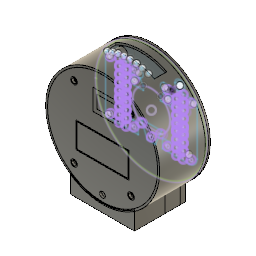
Whatscup design v30 (Autodesk Fusion 360 design; units mm, degrees)
Autodesk Fusion 360 part; units mm, degrees
note: some values were not read from the file. Chosen so that the rebuilt part matches the saved one: which face or edge a step refers to; which pieces of a blend or face edit are solid. Set by a fixed rule: which sketch regions a step uses.
(part 1 of 3)
sketch "Blueprint" plane through (0, 0, 0) normal (0, 1, 0) x (1, 0, 0)
  circle A0 centre (0, 0) radius 17.9
  line L0 (-5.49936, -34.775052) -> (17.60064, -34.775052)
  line L1 (17.60064, -34.775052) -> (17.60064, -22.275052)
  line L2 (17.60064, -22.275052) -> (-5.49936, -22.275052)
  line L3 (-5.49936, -22.275052) -> (-5.49936, -34.775052)
  line L4 (-5.49936, -34.775052) -> (0.00064, -34.775052)
  line L5 (0.00064, -34.775052) -> (0.00064, -22.275052)
  line L6 (0.00064, -22.275052) -> (-5.49936, -22.275052)
  line L7 (-5.49936, -22.275052) -> (-5.49936, -34.775052)
  line L8 (-31.404883, 42.880454) -> (31.412157, 42.880454)
  line L9 (31.412157, 42.880454) -> (31.412157, 63.421004)
  line L10 (31.412157, 63.421004) -> (-31.404883, 63.421004)
  line L11 (-31.404883, 63.421004) -> (-31.404883, 42.880454)
  line L12 (-31.404883, 42.880454) -> (31.412157, 63.421004) construction
  line L13 (31.412157, 42.880454) -> (-31.404883, 63.421004) construction
  circle A1 centre (-28.000001, -35.000001) radius 1.25
  circle A2 centre (28, -35.000001) radius 1.25
  circle A3 centre (27.999999, 34.999999) radius 1.25
  circle A4 centre (-28.000001, 34.999999) radius 1.25
  line L14 (20.00064, -44.468236) -> (-19.99936, -44.468236)
  line L15 (-19.99936, -44.468236) -> (-19.99936, -61.833222)
  line L16 (-19.99936, -61.833222) -> (20.00064, -61.833222)
  line L17 (20.00064, -61.833222) -> (20.00064, -44.468236)
  line L18 (20.00064, -44.468236) -> (-19.99936, -61.833222) construction
  line L19 (-19.99936, -44.468236) -> (20.00064, -61.833222) construction
  circle A5 centre (0, 0) radius 54.966054
  circle A6 centre (0.003637, 48.02163) radius 2.81059
  line L20 (-9.49936, -38.775052) -> (21.60064, -38.775052)
  line L21 (21.60064, -38.775052) -> (21.60064, -18.275052)
  line L22 (21.60064, -18.275052) -> (-9.49936, -18.275052)
  line L23 (-9.49936, -18.275052) -> (-9.49936, -38.775052)
  line L24 (-7.49936, -26.775052) -> (-3.49936, -26.775052)
  line L25 (-3.49936, -26.775052) -> (-3.49936, -30.275052)
  line L26 (-3.49936, -30.275052) -> (-7.49936, -30.275052)
  line L27 (-7.49936, -30.275052) -> (-7.49936, -26.775052)
  line L28 (-7.49936, -26.775052) -> (-3.49936, -30.275052) construction
  line L29 (-3.49936, -26.775052) -> (-7.49936, -30.275052) construction
  circle A7 centre (-28.000001, -35.000001) radius 3.25
  circle A8 centre (-28.000001, 34.999999) radius 3.25
  circle A9 centre (27.999999, 34.999999) radius 3.25
  circle A10 centre (28, -35.000001) radius 1.75
  circle A11 centre (28, -35.000001) radius 2.25
  circle A12 centre (28, -35.000001) radius 3.25
  line L30 (25.06, 21.65) -> (-25.06, 21.65)
  line L31 (-25.06, 21.65) -> (-25.06, -1.65)
  line L32 (-25.06, -1.65) -> (25.06, -1.65)
  line L33 (25.06, -1.65) -> (25.06, 21.65)
  line L34 (25.06, 21.65) -> (-25.06, -1.65) construction
  line L35 (-25.06, 21.65) -> (25.06, -1.65) construction
  line L36 (26.06, 22.65) -> (-26.06, 22.65)
  line L37 (-26.06, 22.65) -> (-26.06, -2.65)
  line L38 (-26.06, -2.65) -> (26.06, -2.65)
  line L39 (26.06, -2.65) -> (26.06, 22.65)
  circle A13 centre (-28.000001, -35.000001) radius 2.25
  circle A14 centre (-28.000001, 34.999999) radius 2.25
  circle A15 centre (27.999999, 34.999999) radius 2.25
  circle A16 centre (0, 0) radius 18.7
  circle A17 centre (39, -25.550001) radius 1.25
  circle A18 centre (39, -25.550001) radius 2.25
  line L40 (25, 7.5) -> (-25, 7.5)
  line L41 (-25, 7.5) -> (-25, -7.5)
  line L42 (-25, -7.5) -> (25, -7.5)
  line L43 (25, -7.5) -> (25, 7.5)
  line L44 (25, 7.5) -> (-25, -7.5) construction
  line L45 (-25, 7.5) -> (25, -7.5) construction
  line L46 (25, 7.5) -> (-25, 7.5)
  line L47 (-25, 7.5) -> (-25, -3)
  line L48 (-25, -3) -> (25, -3)
  line L49 (25, -3) -> (25, 7.5)
  circle A19 centre (39, -25.550001) radius 1.4
  circle A20 centre (0, 0) radius 44.82187 construction
  line L50 (2.50064, -42.32187) -> (-2.49936, -47.32187) construction
  line L51 (-2.49936, -42.32187) -> (2.50064, -47.32187) construction
  circle A21 centre (27.999999, 34.999999) radius 1.35
  circle A22 centre (-28.000001, 34.999999) radius 1.35
  circle A23 centre (-28.000001, -35.000001) radius 1.35
  circle A24 centre (28, -35.000001) radius 1.35
  line L52 (93.409991, -32.672779) -> (81.409991, -32.672779)
  line L53 (81.409991, -32.672779) -> (81.409991, 32.327221)
  line L54 (81.409991, 32.327221) -> (93.409991, 32.327221)
  line L55 (93.409991, 32.327221) -> (93.409991, -32.672779) construction
  line L56 (185, -25) -> (180, -25)
  line L57 (180, -25) -> (180, -20)
  line L58 (180, -20) -> (185, -20)
  line L59 (185, -20) -> (185, -25)
  line L60 (188.500003, -19.05) -> (176.500003, -19.05)
  line L61 (176.500003, -19.05) -> (176.500003, -25.95)
  line L62 (176.500003, -25.95) -> (188.500003, -25.95)
  line L63 (188.500003, -25.95) -> (188.500003, -19.05)
  line L64 (188.500003, -19.05) -> (176.500003, -25.95) construction
  line L65 (176.500003, -19.05) -> (188.500003, -25.95) construction
  line L66 (188.500003, -19.05) -> (176.500003, -25.95) construction
  line L67 (188.500003, -25.95) -> (188.500003, -19.05)
  line L68 (180, -20) -> (185, -20)
  line L69 (180, -25) -> (180, -20)
  line L70 (188.500003, -19.05) -> (176.500003, -19.05)
  line L71 (185, -20) -> (185, -25)
  line L72 (176.500003, -19.05) -> (188.500003, -25.95) construction
  line L73 (176.500003, -19.05) -> (176.500003, -25.95)
  line L74 (185, -25) -> (180, -25)
  line L75 (176.500003, -25.95) -> (188.500003, -25.95)
  line L76 (185, -18.1) -> (180, -18.1)
  line L77 (176.500003, -12.15) -> (188.500003, -19.05) construction
  line L78 (188.500003, -19.05) -> (188.500003, -12.15)
  line L79 (185, -18.1) -> (180, -18.1)
  line L80 (180, -18.1) -> (180, -13.1)
  line L81 (176.500003, -19.05) -> (188.500003, -19.05)
  line L82 (188.500003, -12.15) -> (176.500003, -19.05) construction
  line L83 (185, -13.1) -> (185, -18.1)
  line L84 (176.500003, -19.05) -> (188.500003, -19.05)
  line L85 (180, -13.1) -> (185, -13.1)
  line L86 (188.500003, -12.15) -> (176.500003, -12.15)
  line L87 (185, -13.1) -> (185, -18.1)
  line L88 (188.500003, -12.15) -> (176.500003, -12.15)
  line L89 (188.500003, -19.05) -> (188.500003, -12.15)
  line L90 (176.500003, -12.15) -> (176.500003, -19.05)
  line L91 (180, -13.1) -> (185, -13.1)
  line L92 (180, -18.1) -> (180, -13.1)
  line L93 (176.500003, -12.15) -> (188.500003, -19.05) construction
  line L94 (176.500003, -12.15) -> (176.500003, -19.05)
  line L95 (188.500003, -12.15) -> (176.500003, -19.05) construction
  line L96 (185, -11.2) -> (180, -11.2)
  line L97 (188.500003, -5.25) -> (176.500003, -5.25)
  line L98 (176.500003, -12.15) -> (188.500003, -12.15)
  line L99 (188.500003, -5.25) -> (176.500003, -5.25)
  line L100 (188.500003, -5.25) -> (176.500003, -12.15) construction
  line L101 (188.500003, 1.65) -> (176.500003, 1.65)
  line L102 (185, -4.3) -> (180, -4.3)
  line L103 (176.500003, -5.25) -> (176.500003, -12.15)
  line L104 (176.500003, 1.65) -> (176.500003, -5.25)
  line L105 (188.500003, -12.15) -> (188.500003, -5.25)
  line L106 (176.500003, -5.25) -> (188.500003, -5.25)
  line L107 (176.500003, -5.25) -> (188.500003, -12.15) construction
  line L108 (176.500003, -5.25) -> (188.500003, -12.15) construction
  line L109 (180, -11.2) -> (180, -6.2)
  line L110 (185, -6.2) -> (185, -11.2)
  line L111 (180, 0.7) -> (185, 0.7)
  line L112 (185, 0.7) -> (185, -4.3)
  line L113 (176.500003, 1.65) -> (188.500003, -5.25) construction
  line L114 (188.500003, -5.25) -> (188.500003, 1.65)
  line L115 (180, -6.2) -> (185, -6.2)
  line L116 (188.500003, 1.65) -> (176.500003, -5.25) construction
  line L117 (180, -11.2) -> (180, -6.2)
  line L118 (176.500003, -5.25) -> (188.500003, -5.25)
  line L119 (180, -4.3) -> (180, 0.7)
  line L120 (188.500003, 1.65) -> (176.500003, -5.25) construction
  line L121 (185, -11.2) -> (180, -11.2)
  line L122 (176.500003, -12.15) -> (188.500003, -12.15)
  line L123 (176.500003, 1.65) -> (188.500003, -5.25) construction
  line L124 (188.500003, 1.65) -> (176.500003, 1.65)
  line L125 (185, -4.3) -> (180, -4.3)
  line L126 (180, -6.2) -> (185, -6.2)
  line L127 (176.500003, 1.65) -> (176.500003, -5.25)
  line L128 (188.500003, -5.25) -> (188.500003, 1.65)
  line L129 (185, -6.2) -> (185, -11.2)
  line L130 (176.500003, -5.25) -> (176.500003, -12.15)
  line L131 (185, 0.7) -> (185, -4.3)
  line L132 (188.500003, -12.15) -> (188.500003, -5.25)
  line L133 (188.500003, -5.25) -> (176.500003, -12.15) construction
  line L134 (180, 0.7) -> (185, 0.7)
  line L135 (180, -4.3) -> (180, 0.7)
  line L136 (176.500003, 15.45) -> (188.500003, 8.55) construction
  line L137 (180, 9.5) -> (180, 14.5)
  line L138 (185, 23.3) -> (180, 23.3)
  line L139 (188.500003, 22.35) -> (176.500003, 22.35)
  line L140 (180, 16.4) -> (180, 21.4)
  line L141 (180, 21.4) -> (185, 21.4)
  line L142 (185, 16.4) -> (180, 16.4)
  line L143 (176.500003, 22.35) -> (188.500003, 15.45) construction
  line L144 (176.500003, 15.45) -> (188.500003, 15.45)
  line L145 (180, 28.3) -> (185, 28.3)
  line L146 (188.500003, 29.25) -> (176.500003, 22.35) construction
  line L147 (188.500003, 22.35) -> (176.500003, 22.35)
  line L148 (188.500003, 8.55) -> (176.500003, 8.55)
  line L149 (185, 2.6) -> (180, 2.6)
  line L150 (180, 2.6) -> (180, 7.6)
  line L151 (185, 2.6) -> (180, 2.6)
  line L152 (180, 9.5) -> (180, 14.5)
  line L153 (180, 7.6) -> (185, 7.6)
  line L154 (176.500003, 1.65) -> (188.500003, 1.65)
  line L155 (180, 14.5) -> (185, 14.5)
  line L156 (188.500003, 15.45) -> (176.500003, 8.55) construction
  line L157 (185, 7.6) -> (185, 2.6)
  line L158 (185, 7.6) -> (185, 2.6)
  line L159 (185, 21.4) -> (185, 16.4)
  line L160 (188.500003, 1.65) -> (188.500003, 8.55)
  line L161 (188.500003, 22.35) -> (188.500003, 29.25)
  line L162 (185, 14.5) -> (185, 9.5)
  line L163 (188.500003, 8.55) -> (188.500003, 15.45)
  line L164 (185, 28.3) -> (185, 23.3)
  line L165 (188.500003, 15.45) -> (188.500003, 22.35)
  line L166 (185, 21.4) -> (185, 16.4)
  line L167 (188.500003, 1.65) -> (188.500003, 8.55)
  line L168 (180, 23.3) -> (180, 28.3)
  line L169 (185, 23.3) -> (180, 23.3)
  line L170 (176.500003, 15.45) -> (188.500003, 15.45)
  line L171 (176.500003, 22.35) -> (188.500003, 15.45) construction
  line L172 (188.500003, 8.55) -> (188.500003, 15.45)
  line L173 (188.500003, 29.25) -> (176.500003, 29.25)
  line L174 (188.500003, 29.25) -> (176.500003, 29.25)
  line L175 (185, 16.4) -> (180, 16.4)
  line L176 (180, 28.3) -> (185, 28.3)
  line L177 (185, 14.5) -> (185, 9.5)
  line L178 (185, 28.3) -> (185, 23.3)
  line L179 (188.500003, 22.35) -> (188.500003, 29.25)
  line L180 (188.500003, 15.45) -> (188.500003, 22.35)
  line L181 (180, 23.3) -> (180, 28.3)
  line L182 (176.500003, 22.35) -> (188.500003, 22.35)
  line L183 (176.500003, 29.25) -> (188.500003, 22.35) construction
  line L184 (188.500003, 22.35) -> (176.500003, 15.45) construction
  line L185 (180, 21.4) -> (185, 21.4)
  line L186 (176.500003, 22.35) -> (188.500003, 22.35)
  line L187 (180, 16.4) -> (180, 21.4)
  line L188 (176.500003, 29.25) -> (188.500003, 22.35) construction
  line L189 (188.500003, 22.35) -> (176.500003, 15.45) construction
  line L190 (188.500003, 29.25) -> (176.500003, 22.35) construction
  line L191 (180, 2.6) -> (180, 7.6)
  line L192 (176.500003, 1.65) -> (188.500003, 1.65)
  line L193 (188.500003, 15.45) -> (176.500003, 15.45)
  line L194 (185, 9.5) -> (180, 9.5)
  line L195 (176.500003, 29.25) -> (176.500003, 22.35)
  line L196 (176.500003, 22.35) -> (176.500003, 15.45)
  line L197 (176.500003, 29.25) -> (176.500003, 22.35)
  line L198 (176.500003, 22.35) -> (176.500003, 15.45)
  line L199 (176.500003, 15.45) -> (176.500003, 8.55)
  line L200 (176.500003, 15.45) -> (176.500003, 8.55)
  line L201 (176.500003, 8.55) -> (176.500003, 1.65)
  line L202 (176.500003, 8.55) -> (176.500003, 1.65)
  line L203 (176.500003, 15.45) -> (188.500003, 8.55) construction
  line L204 (188.500003, 15.45) -> (176.500003, 8.55) construction
  line L205 (176.500003, 8.55) -> (188.500003, 8.55)
  line L206 (180, 7.6) -> (185, 7.6)
  line L207 (180, 14.5) -> (185, 14.5)
  line L208 (188.500003, 8.55) -> (176.500003, 8.55)
  line L209 (188.500003, 15.45) -> (176.500003, 15.45)
  line L210 (176.500003, 8.55) -> (188.500003, 1.65) construction
  line L211 (176.500003, 8.55) -> (188.500003, 8.55)
  line L212 (188.500003, 8.55) -> (176.500003, 1.65) construction
  line L213 (188.500003, 8.55) -> (176.500003, 1.65) construction
  line L214 (185, 9.5) -> (180, 9.5)
  line L215 (176.500003, 8.55) -> (188.500003, 1.65) construction
  line L216 (25.499998, -0.45) -> (25.499998, 4.55)
  line L217 (22, 19.299999) -> (34, 12.399999) construction
  line L218 (30.499998, 13.35) -> (25.499998, 13.35)
  line L219 (25.499998, 6.45) -> (25.499998, 11.45)
  line L220 (25.499998, 11.45) -> (30.499998, 11.45)
  line L221 (22, 26.199999) -> (34, 19.299999) construction
  line L222 (25.499998, 18.35) -> (30.499998, 18.35)
  line L223 (25.499998, 25.25) -> (30.499998, 25.25)
  line L224 (22, 5.499999) -> (34, -1.400001) construction
  line L225 (22, 12.399999) -> (34, 5.499999) construction
  line L226 (22, -1.400001) -> (34, -8.300001) construction
  line L227 (25.499998, -7.35) -> (25.499998, -2.35)
  line L228 (25.499998, 18.35) -> (30.499998, 18.35)
  line L229 (30.499998, 20.25) -> (25.499998, 20.25)
  line L230 (34, -1.400001) -> (22, -8.300001) construction
  line L231 (30.499998, -0.45) -> (25.499998, -0.45)
  line L232 (22, -1.400001) -> (34, -8.300001) construction
  line L233 (22, 12.399999) -> (34, 5.499999) construction
  line L234 (30.499998, 25.25) -> (30.499998, 20.25)
  line L235 (30.499998, -9.25) -> (30.499998, -14.25)
  line L236 (30.499998, -2.35) -> (30.499998, -7.35)
  line L237 (30.499998, 18.35) -> (30.499998, 13.35)
  line L238 (30.499998, -16.15) -> (30.499998, -21.15)
  line L239 (30.499998, -23.05) -> (30.499998, -28.05)
  line L240 (30.499998, 18.35) -> (30.499998, 13.35)
  line L241 (30.499998, 25.25) -> (30.499998, 20.25)
  line L242 (30.499998, -2.35) -> (30.499998, -7.35)
  line L243 (30.499998, -16.15) -> (30.499998, -21.15)
  line L244 (25.499998, -16.15) -> (30.499998, -16.15)
  line L245 (30.499998, -28.05) -> (25.499998, -28.05)
  line L246 (25.499998, -14.25) -> (25.499998, -9.25)
  line L247 (25.499998, -2.35) -> (30.499998, -2.35)
  line L248 (30.499998, -21.15) -> (25.499998, -21.15)
  line L249 (30.499998, -7.35) -> (25.499998, -7.35)
  line L250 (34, -1.400001) -> (22, -8.300001) construction
  line L251 (25.499998, -7.35) -> (25.499998, -2.35)
  line L252 (30.499998, -0.45) -> (25.499998, -0.45)
  line L253 (34, 12.399999) -> (22, 5.499999) construction
  line L254 (30.499998, 20.25) -> (25.499998, 20.25)
  line L255 (22, -15.200001) -> (34, -22.100001) construction
  line L256 (22, -22.100001) -> (34, -22.100001)
  line L257 (22, -15.200001) -> (34, -15.200001)
  line L258 (22, -15.200001) -> (34, -22.100001) construction
  line L259 (25.499998, -14.25) -> (25.499998, -9.25)
  line L260 (30.499998, -14.25) -> (25.499998, -14.25)
  line L261 (25.499998, -28.05) -> (25.499998, -23.05)
  line L262 (34, -8.300001) -> (22, -15.200001) construction
  line L263 (22, -8.300001) -> (34, -15.200001) construction
  line L264 (25.499998, -16.15) -> (30.499998, -16.15)
  line L265 (30.499998, 6.45) -> (25.499998, 6.45)
  line L266 (30.499998, 11.45) -> (30.499998, 6.45)
  line L267 (25.499998, -0.45) -> (25.499998, 4.55)
  line L268 (30.499998, 4.55) -> (30.499998, -0.45)
  line L269 (34, 19.299999) -> (22, 12.399999) construction
  line L270 (30.499998, -9.25) -> (30.499998, -14.25)
  line L271 (25.499998, 4.55) -> (30.499998, 4.55)
  line L272 (30.499998, -23.05) -> (30.499998, -28.05)
  line L273 (30.499998, 11.45) -> (30.499998, 6.45)
  line L274 (34, 5.499999) -> (22, -1.400001) construction
  line L275 (30.499998, 4.55) -> (30.499998, -0.45)
  line L276 (22, -15.200001) -> (34, -15.200001)
  line L277 (22, -8.300001) -> (34, -15.200001) construction
  line L278 (25.499998, -23.05) -> (30.499998, -23.05)
  line L279 (25.499998, -21.15) -> (25.499998, -16.15)
  line L280 (34, 12.399999) -> (22, 5.499999) construction
  line L281 (30.499998, 6.45) -> (25.499998, 6.45)
  line L282 (22, -22.100001) -> (34, -29.000001) construction
  line L283 (34, 26.199999) -> (22, 19.299999) construction
  line L284 (30.499998, 13.35) -> (25.499998, 13.35)
  line L285 (34, -15.200001) -> (22, -22.100001) construction
  line L286 (25.499998, -9.25) -> (30.499998, -9.25)
  line L287 (25.499998, 6.45) -> (25.499998, 11.45)
  line L288 (25.499998, -9.25) -> (30.499998, -9.25)
  line L289 (25.499998, -28.05) -> (25.499998, -23.05)
  line L290 (30.499998, -28.05) -> (25.499998, -28.05)
  line L291 (34, 19.299999) -> (22, 12.399999) construction
  line L292 (25.499998, 25.25) -> (30.499998, 25.25)
  line L293 (25.499998, 13.35) -> (25.499998, 18.35)
  line L294 (34, -8.300001) -> (22, -15.200001) construction
  line L295 (25.499998, -2.35) -> (30.499998, -2.35)
  line L296 (22, 5.499999) -> (34, -1.400001) construction
  line L297 (25.499998, -23.05) -> (30.499998, -23.05)
  line L298 (25.499998, 13.35) -> (25.499998, 18.35)
  line L299 (25.499998, 20.25) -> (25.499998, 25.25)
  line L300 (25.499998, -21.15) -> (25.499998, -16.15)
  line L301 (30.499998, -14.25) -> (25.499998, -14.25)
  line L302 (34, 26.199999) -> (22, 19.299999) construction
  line L303 (30.499998, -7.35) -> (25.499998, -7.35)
  line L304 (34, -22.100001) -> (22, -29.000001) construction
  line L305 (34, 5.499999) -> (22, -1.400001) construction
  line L306 (34, -15.200001) -> (22, -22.100001) construction
  line L307 (30.499998, -21.15) -> (25.499998, -21.15)
  line L308 (22, 26.199999) -> (34, 19.299999) construction
  line L309 (25.499998, 20.25) -> (25.499998, 25.25)
  line L310 (22, 19.299999) -> (34, 12.399999) construction
  line L311 (34, -22.100001) -> (22, -29.000001) construction
  line L312 (22, -22.100001) -> (34, -29.000001) construction
  line L313 (25.499998, 11.45) -> (30.499998, 11.45)
  line L314 (25.499998, 4.55) -> (30.499998, 4.55)
  line L315 (28, -35.000001) -> (27.999999, 34.999999)
  line L316 (-28.000001, -35.000001) -> (-28.000001, 34.999999) construction
  line L317 (28, -29.000001) -> (28, -22.100001) construction
  circle A25 centre (16, -25.550001) radius 2.25
  circle A26 centre (16, -25.550001) radius 1.25
  circle A27 centre (16, -25.550001) radius 1.4
  circle A28 centre (39, 22.749999) radius 1.25
  circle A29 centre (39, 22.749999) radius 2.25
  circle A30 centre (39, 22.749999) radius 1.4
  line L318 (39, -25.550001) -> (39, 29) construction
  line L319 (39, 22.749999) -> (-2.19113, 22.749999) construction
  circle A31 centre (16, 22.749999) radius 1.25
  circle A32 centre (16, 22.749999) radius 1.4
  circle A33 centre (16, 22.749999) radius 2.25
  line L320 (30.649998, 13.2) -> (25.349998, 13.2)
  line L321 (25.349998, 13.2) -> (25.349998, 18.5)
  line L322 (25.349998, 18.5) -> (30.649998, 18.5)
  line L323 (30.649998, 18.5) -> (30.649998, 13.2)
  line L324 (30.649998, -0.6) -> (25.349998, -0.6)
  line L325 (25.349998, -0.6) -> (25.349998, 4.7)
  line L326 (25.349998, 4.7) -> (30.649998, 4.7)
  line L327 (30.649998, 4.7) -> (30.649998, -0.6)
  line L328 (30.649998, -9.1) -> (30.649998, -14.4)
  line L329 (30.649998, -14.4) -> (25.349998, -14.4)
  line L330 (25.349998, -14.4) -> (25.349998, -9.1)
  line L331 (25.349998, -9.1) -> (30.649998, -9.1)
  line L332 (30.649998, -21.3) -> (25.349998, -21.3)
  line L333 (25.349998, -21.3) -> (25.349998, -16)
  line L334 (25.349998, -16) -> (30.649998, -16)
  line L335 (30.649998, -16) -> (30.649998, -21.3)
  line L336 (30.649998, -28.2) -> (25.349998, -28.2)
  line L337 (25.349998, -28.2) -> (25.349998, -22.9)
  line L338 (25.349998, -22.9) -> (30.649998, -22.9)
  line L339 (30.649998, -22.9) -> (30.649998, -28.2)
  line L340 (22, -15.050001) -> (34, -15.050001) construction
  line L341 (30.649998, -7.5) -> (25.349998, -7.5)
  line L342 (25.349998, -7.5) -> (25.349998, -2.2)
  line L343 (25.349998, -2.2) -> (30.649998, -2.2)
  line L344 (30.649998, -2.2) -> (30.649998, -7.5)
  line L345 (30.649998, 6.3) -> (25.349998, 6.3)
  line L346 (25.349998, 6.3) -> (25.349998, 11.6)
  line L347 (25.349998, 11.6) -> (30.649998, 11.6)
  line L348 (30.649998, 11.6) -> (30.649998, 6.3)
  line L349 (30.649998, 20.1) -> (25.349998, 20.1)
  line L350 (25.349998, 20.1) -> (25.349998, 25.4)
  line L351 (25.349998, 25.4) -> (30.649998, 25.4)
  line L352 (30.649998, 25.4) -> (30.649998, 20.1)
  circle A34 centre (-40, -25.550001) radius 1.25
  circle A35 centre (-40, -25.550001) radius 1.4
  circle A36 centre (-40, -25.550001) radius 2.25
  circle A37 centre (-17, -25.550001) radius 2.25
  circle A38 centre (-17, -25.550001) radius 1.4
  circle A39 centre (-17, -25.550001) radius 1.25
  line L353 (-24.600002, -28.95) -> (-31.400002, -28.95)
  line L354 (-31.400002, -28.95) -> (-31.400002, -22.15)
  line L355 (-31.400002, -22.15) -> (-24.600002, -22.15)
  line L356 (-24.600002, -22.15) -> (-24.600002, -28.95)
  line L357 (-30.650002, -22.9) -> (-25.350002, -22.9)
  line L358 (-30.500002, -23.05) -> (-25.500002, -23.05)
  line L359 (-25.500002, -23.05) -> (-25.500002, -28.05)
  line L360 (-25.350002, -22.9) -> (-25.350002, -28.2)
  line L361 (-30.500002, -28.05) -> (-30.500002, -23.05)
  line L362 (-30.650002, -28.2) -> (-30.650002, -22.9)
  line L363 (-25.350002, -28.2) -> (-30.650002, -28.2)
  line L364 (-25.500002, -28.05) -> (-30.500002, -28.05)
  line L365 (-24.600002, -22.05) -> (-31.400002, -22.05)
  line L366 (-31.400002, -22.05) -> (-31.400002, -15.25)
  line L367 (-24.600002, -15.25) -> (-24.600002, -22.05)
  line L368 (-25.350002, -21.3) -> (-30.650002, -21.3)
  line L369 (-25.500002, -21.15) -> (-30.500002, -21.15)
  line L370 (-30.500002, -21.15) -> (-30.500002, -16.15)
  line L371 (-30.650002, -21.3) -> (-30.650002, -16)
  line L372 (-25.500002, -16.15) -> (-25.500002, -21.15)
  line L373 (-25.350002, -16) -> (-25.350002, -21.3)
  line L374 (-30.500002, -16.15) -> (-25.500002, -16.15)
  line L375 (-30.650002, -16) -> (-25.350002, -16)
  line L376 (-31.400002, -15.25) -> (-24.600002, -15.25)
  line L377 (-24.600002, -15.15) -> (-31.400002, -15.15)
  line L378 (-31.400002, -15.15) -> (-31.400002, -8.35)
  line L379 (-24.600002, -8.35) -> (-24.600002, -15.15)
  line L380 (-25.350002, -14.4) -> (-30.650002, -14.4)
  line L381 (-25.500002, -14.25) -> (-30.500002, -14.25)
  line L382 (-25.500002, -9.25) -> (-25.500002, -14.25)
  line L383 (-25.350002, -9.1) -> (-25.350002, -14.4)
  line L384 (-30.500002, -14.25) -> (-30.500002, -9.25)
  line L385 (-30.650002, -14.4) -> (-30.650002, -9.1)
  line L386 (-30.500002, -9.25) -> (-25.500002, -9.25)
  line L387 (-30.650002, -9.1) -> (-25.350002, -9.1)
  line L388 (-31.400002, -8.35) -> (-24.600002, -8.35)
  line L389 (-24.600002, -8.25) -> (-31.400002, -8.25)
  line L390 (-31.400002, -8.25) -> (-31.400002, -1.45)
  line L391 (-25.350002, -7.5) -> (-30.650002, -7.5)
  line L392 (-25.500002, -7.35) -> (-30.500002, -7.35)
  line L393 (-30.650002, -7.5) -> (-30.650002, -2.2)
  line L394 (-30.500002, -7.35) -> (-30.500002, -2.35)
  line L395 (-25.500002, -2.35) -> (-25.500002, -7.35)
  line L396 (-25.350002, -2.2) -> (-25.350002, -7.5)
  line L397 (-24.600002, -1.45) -> (-24.600002, -8.25)
  line L398 (-30.500002, -2.35) -> (-25.500002, -2.35)
  line L399 (-30.650002, -2.2) -> (-25.350002, -2.2)
  line L400 (-31.400002, -1.45) -> (-24.600002, -1.45)
  line L401 (-24.600002, -1.35) -> (-31.400002, -1.35)
  line L402 (-31.400002, -1.35) -> (-31.400002, 2.966827)
  line L403 (-30.650002, -0.6) -> (-30.650002, 4.7)
  line L404 (-25.350002, -0.6) -> (-30.650002, -0.6)
  line L405 (-25.500002, 4.55) -> (-25.500002, -0.45)
  line L406 (-25.350002, 4.7) -> (-25.350002, -0.6)
  line L407 (-24.600002, 1.133176) -> (-24.600002, -0.943173)
  line L408 (-24.600002, -0.943173) -> (-24.600002, -1.35)
  line L409 (-25.500002, -0.45) -> (-30.500002, -0.45)
  line L410 (-30.500002, -0.45) -> (-30.500002, 4.55)
  line L411 (-24.600002, 5.45) -> (-24.600002, 1.133176)
  line L412 (-31.400002, 2.966827) -> (-31.400002, 5.043176)
  line L413 (-30.500002, 4.55) -> (-25.500002, 4.55)
  line L414 (-30.650002, 4.7) -> (-25.350002, 4.7)
  line L415 (-31.400002, 5.45) -> (-24.600002, 5.45)
  line L416 (-24.600002, 5.55) -> (-31.400002, 5.55)
  line L417 (-31.400002, 5.043176) -> (-31.400002, 5.45)
  line L418 (-31.400002, 5.55) -> (-31.400002, 12.35)
  line L419 (-25.350002, 6.3) -> (-30.650002, 6.3)
  line L420 (-25.350002, 11.6) -> (-25.350002, 6.3)
  line L421 (-25.500002, 11.45) -> (-25.500002, 6.45)
  line L422 (-25.500002, 6.45) -> (-30.500002, 6.45)
  line L423 (-24.600002, 12.35) -> (-24.600002, 5.55)
  line L424 (-30.500002, 6.45) -> (-30.500002, 11.45)
  line L425 (-30.650002, 6.3) -> (-30.650002, 11.6)
  line L426 (-30.500002, 11.45) -> (-25.500002, 11.45)
  line L427 (-30.650002, 11.6) -> (-25.350002, 11.6)
  line L428 (-31.400002, 12.35) -> (-24.600002, 12.35)
  line L429 (-24.600002, 12.45) -> (-31.400002, 12.45)
  line L430 (-31.400002, 12.45) -> (-31.400002, 19.25)
  line L431 (-25.350002, 13.2) -> (-30.650002, 13.2)
  line L432 (-30.650002, 13.2) -> (-30.650002, 18.5)
  line L433 (-25.500002, 13.35) -> (-30.500002, 13.35)
  line L434 (-30.500002, 13.35) -> (-30.500002, 18.35)
  line L435 (-25.500002, 18.35) -> (-25.500002, 13.35)
  line L436 (-25.350002, 18.5) -> (-25.350002, 13.2)
  line L437 (-24.600002, 19.25) -> (-24.600002, 12.45)
  line L438 (-30.500002, 18.35) -> (-25.500002, 18.35)
  line L439 (-30.650002, 18.5) -> (-25.350002, 18.5)
  line L440 (-31.400002, 19.25) -> (-24.600002, 19.25)
  line L441 (-24.600002, 19.35) -> (-31.400002, 19.35)
  line L442 (-31.400002, 19.35) -> (-31.400002, 26.15)
  line L443 (-25.350002, 20.1) -> (-30.650002, 20.1)
  line L444 (-30.650002, 20.1) -> (-30.650002, 25.4)
  line L445 (-30.500002, 20.25) -> (-30.500002, 25.25)
  line L446 (-25.500002, 20.25) -> (-30.500002, 20.25)
  line L447 (-25.500002, 25.25) -> (-25.500002, 20.25)
  line L448 (-25.350002, 25.4) -> (-25.350002, 20.1)
  line L449 (-24.600002, 26.15) -> (-24.600002, 19.35)
  line L450 (-30.500002, 25.25) -> (-25.500002, 25.25)
  line L451 (-30.650002, 25.4) -> (-25.350002, 25.4)
  line L452 (-31.400002, 26.15) -> (-24.600002, 26.15)
  circle A40 centre (-40, 22.749999) radius 1.4
  circle A41 centre (-40, 22.749999) radius 1.25
  circle A42 centre (-40, 22.749999) radius 2.25
  circle A43 centre (-17, 22.749999) radius 2.25
  circle A44 centre (-17, 22.749999) radius 1.4
  circle A45 centre (-17, 22.749999) radius 1.25
  circle A46 centre (0, 0) radius 18.05
  line L453 (0, 0) -> (0, 20) construction
  line L454 (9, 15.472879) -> (-9, 15.472879)
  line L455 (31.399998, 12.45) -> (24.599998, 12.45)
  line L456 (24.599998, 12.45) -> (24.599998, 19.25)
  line L457 (24.599998, 19.25) -> (31.399998, 19.25)
  line L458 (31.399998, 19.25) -> (31.399998, 12.45)
  line L459 (24.599998, -1.45) -> (31.399998, -1.45)
  line L460 (31.399998, -1.45) -> (31.399998, -8.25)
  line L461 (31.399998, -8.25) -> (24.599998, -8.25)
  line L462 (24.599998, -8.25) -> (24.599998, -1.45)
  line L463 (31.399998, -15.25) -> (31.399998, -22.05)
  line L464 (31.399998, -22.05) -> (24.599998, -22.05)
  line L465 (24.599998, -22.05) -> (24.599998, -15.25)
  line L466 (24.599998, -15.25) -> (31.399998, -15.25)
  line L467 (24.599998, -28.95) -> (24.599998, -22.15)
  line L468 (24.599998, -22.15) -> (31.399998, -22.15)
  line L469 (31.399998, -22.15) -> (31.399998, -28.95)
  line L470 (31.399998, -28.95) -> (24.599998, -28.95)
  line L471 (31.399998, -15.15) -> (24.599998, -15.15)
  line L472 (24.599998, -15.15) -> (24.599998, -8.35)
  line L473 (24.599998, -8.35) -> (31.399998, -8.35)
  line L474 (31.399998, -8.35) -> (31.399998, -15.15)
  line L475 (24.599998, 5.043176) -> (31.399998, 1.133176) construction
  line L476 (31.399998, 1.133176) -> (34.448624, -0.619785) construction
  arc A47 (33.551376, -2.180216) -> (34.448624, -0.619785) centre (34, -1.400001) ccw construction
  line L477 (31.399998, -0.943173) -> (33.551376, -2.180216) construction
  line L478 (31.399998, 1.133176) -> (31.399998, -0.943173)
  line L479 (24.599998, 2.966827) -> (24.599998, 5.043176)
  line L480 (24.599998, 5.043176) -> (24.599998, 5.45)
  line L481 (24.599998, 5.45) -> (31.399998, 5.45)
  line L482 (31.399998, 5.45) -> (31.399998, 1.133176)
  line L483 (31.399998, -0.943173) -> (31.399998, -1.35)
  line L484 (31.399998, -1.35) -> (24.599998, -1.35)
  line L485 (24.599998, -1.35) -> (24.599998, 2.966827)
  line L486 (21.551376, 4.719784) -> (24.599998, 2.966827) construction
  arc A48 (22.448624, 6.280215) -> (21.551376, 4.719784) centre (22, 5.499999) ccw construction
  line L487 (22.448624, 6.280215) -> (24.599998, 5.043176) construction
  line L488 (24.599998, 2.966827) -> (31.399998, -0.943173) construction
  line L489 (31.399998, 5.55) -> (24.599998, 5.55)
  line L490 (24.599998, 5.55) -> (24.599998, 12.35)
  line L491 (24.599998, 12.35) -> (31.399998, 12.35)
  line L492 (31.399998, 12.35) -> (31.399998, 5.55)
  line L493 (31.399998, 26.15) -> (31.399998, 19.35)
  line L494 (31.399998, 19.35) -> (24.599998, 19.35)
  line L495 (24.599998, 19.35) -> (24.599998, 26.15)
  line L496 (24.599998, 26.15) -> (31.399998, 26.15)
  line L497 (9, 15.472879) -> (11.1, 15.472879)
  line L498 (-9, 15.472879) -> (-10.8, 15.472879)
  line L499 (-9.294757, 15.472879) -> (-10.501428, 15.472879)
  circle A49 centre (0, 22.749999) radius 2.25
  circle A50 centre (0, 22.749999) radius 1.25
  circle A51 centre (0, 22.749999) radius 1.4
  circle A52 centre (-17, -17.550001) radius 1.25
  circle A53 centre (-17, -17.550001) radius 1.4
  circle A54 centre (-17, -17.550001) radius 2.25
  circle A55 centre (16, -17.550001) radius 1.25
  circle A56 centre (16, -17.550001) radius 1.4
  circle A57 centre (16, -17.550001) radius 2.25
  point P0 (0.003637, 53.150729)
  point P1 (0.00064, -53.150729)
  point P2 (-5.49936, -28.525052)
  point P3 (0, 10)
  point P4 (0.00064, -44.82187)
  point P5 (182.500003, -22.5)
  point P6 (182.500003, -22.5)
  point P7 (182.500003, -15.6)
  point P8 (182.500003, -15.6)
  point P9 (182.500003, -1.8)
  point P10 (182.500003, -1.8)
  point P11 (182.500003, -8.7)
  point P12 (182.500003, -8.7)
  point P13 (182.500003, 25.8)
  point P14 (182.500003, 18.9)
  point P15 (182.500003, 25.8)
  point P16 (182.500003, 18.9)
  point P17 (182.500003, 12)
  point P18 (182.500003, 12)
  point P19 (182.500003, 5.1)
  point P20 (182.500003, 5.1)
  point P21 (28, -4.850001)
  point P22 (28, -11.750001)
  point P23 (28, -4.850001)
  point P24 (28, -11.750001)
  point P25 (28, 22.749999)
  point P26 (28, 15.849999)
  point P27 (28, 22.749999)
  point P28 (28, -18.650001)
  point P29 (28, -18.650001)
  point P30 (28, -25.550001)
  point P31 (28, 8.949999)
  point P32 (28, 15.849999)
  point P33 (28, 8.949999)
  point P34 (28, 2.049999)
  point P35 (28, 2.049999)
  point P36 (28, -25.550001)
  point P37 (16.732262, -25.825445)
  point P38 (39.732262, 22.174555)
  dimension "d1" = 35.8
  dimension "d4" = 23.1
  dimension "d5" = 12.5
  dimension "d6" = 5.5
  dimension "d7" = 12.5
  dimension "d9" = 2.5
  dimension "d10" = 2.5
  dimension "d11" = 2.5
  dimension "d12" = 2.5
  dimension "d13" = 40
  dimension "d43" = 5.62118
  dimension "d44" = 4
  dimension "d47" = 4
  dimension "d48" = 3.5
  dimension "d69" = 2
  dimension "d70" = 2
  dimension "d71" = 2
  dimension "d104" = 3.5
  dimension "d105" = 4.5
  dimension "d106" = 6.5
  dimension "d136" = 50.12
  dimension "d137" = 23.3
  dimension "d138" = 1
  dimension "d145" = 4.5
  dimension "d146" = 4.5
  dimension "d147" = 4.5
  dimension "d154" = 37.4
  dimension "d157" = 2.5
  dimension "d158" = 4.5
  dimension "d159" = 50
  dimension "d160" = 15
  dimension "d161" = 50
  dimension "d162" = 10.5
  dimension "d169" = 0.15
  dimension "d174" = 5
  dimension "d175" = 5
  dimension "d184" = 2.7
  dimension "d187" = 2.7
  dimension "d188" = 2.7
  dimension "d189" = 2.7
  dimension "d213" = 12
  dimension "d214" = 65
  dimension "d215" = 5
  dimension "d216" = 5
  dimension "d219" = 12
  dimension "d220" = 6.9
  dimension "d221" = 5
  dimension "d222" = 5
  dimension "d223" = 12
  dimension "d224" = 6.9
  dimension "d225" = 5
  dimension "d226" = 5
  dimension "d227" = 12
  dimension "d228" = 6.9
  dimension "d229" = 5
  dimension "d230" = 5
  dimension "d231" = 12
  dimension "d232" = 6.9
  dimension "d233" = 5
  dimension "d234" = 5
  dimension "d235" = 12
  dimension "d236" = 6.9
  dimension "d237" = 5
  dimension "d238" = 5
  dimension "d239" = 12
  dimension "d240" = 6.9
  dimension "d241" = 5
  dimension "d242" = 5
  dimension "d243" = 12
  dimension "d244" = 6.9
  dimension "d245" = 5
  dimension "d246" = 5
  dimension "d247" = 12
  dimension "d248" = 6.9
  dimension "d249" = 5
  dimension "d250" = 5
  dimension "d251" = 12
  dimension "d252" = 6.9
  dimension "d253" = 5
  dimension "d254" = 5
  dimension "d255" = 12
  dimension "d256" = 6.9
  dimension "d257" = 5
  dimension "d258" = 5
  dimension "d259" = 12
  dimension "d260" = 6.9
  dimension "d261" = 5
  dimension "d262" = 5
  dimension "d263" = 12
  dimension "d264" = 6.9
  dimension "d265" = 5
  dimension "d266" = 5
  dimension "d267" = 12
  dimension "d268" = 6.9
  dimension "d269" = 5
  dimension "d270" = 5
  dimension "d271" = 12
  dimension "d272" = 6.9
  dimension "d273" = 5
  dimension "d274" = 5
  dimension "d275" = 12
  dimension "d276" = 6.9
  dimension "d277" = 5
  dimension "d278" = 5
  dimension "d279" = 12
  dimension "d280" = 6.9
  dimension "d281" = 55.2
  dimension "d282" = 5
  dimension "d283" = 5
  dimension "d284" = 12
  dimension "d285" = 6.9
  dimension "d286" = 5
  dimension "d287" = 5
  dimension "d288" = 12
  dimension "d289" = 6.9
  dimension "d290" = 5
  dimension "d291" = 5
  dimension "d292" = 12
  dimension "d293" = 6.9
  dimension "d294" = 5
  dimension "d295" = 5
  dimension "d296" = 12
  dimension "d297" = 6.9
  dimension "d298" = 5
  dimension "d299" = 5
  dimension "d300" = 12
  dimension "d301" = 6.9
  dimension "d302" = 5
  dimension "d303" = 5
  dimension "d304" = 12
  dimension "d305" = 6.9
  dimension "d306" = 5
  dimension "d307" = 5
  dimension "d308" = 12
  dimension "d309" = 6.9
  dimension "d310" = 5
  dimension "d311" = 5
  dimension "d312" = 12
  dimension "d313" = 6.9
  dimension "d314" = 5
  dimension "d315" = 5
  dimension "d316" = 12
  dimension "d317" = 6.9
  dimension "d318" = 5
  dimension "d319" = 5
  dimension "d320" = 12
  dimension "d321" = 6.9
  dimension "d322" = 5
  dimension "d323" = 5
  dimension "d324" = 12
  dimension "d325" = 6.9
  dimension "d326" = 5
  dimension "d327" = 5
  dimension "d328" = 12
  dimension "d329" = 6.9
  dimension "d330" = 5
  dimension "d331" = 5
  dimension "d332" = 12
  dimension "d333" = 6.9
  dimension "d334" = 5
  dimension "d335" = 5
  dimension "d336" = 12
  dimension "d337" = 6.9
  dimension "d338" = 5
  dimension "d339" = 5
  dimension "d340" = 12
  dimension "d341" = 6.9
  dimension "d342" = 5
  dimension "d343" = 5
  dimension "d344" = 12
  dimension "d345" = 6.9
  dimension "d346" = 55.2
  dimension "d347" = 0.15
  dimension "d348" = 2.5
  dimension "d349" = 4.5
  dimension "d350" = 0.15
  dimension "d352" = 2.5
  dimension "d353" = 4.5
  dimension "d356" = 0.15
  dimension "d357" = 2.5
  dimension "d358" = 4.5
  dimension "d359" = -0.15
  dimension "d360" = -0.9
  dimension "d361" = 0.15
  dimension "d362" = 0.15
  dimension "d363" = 0.15
  dimension "d364" = 0.15
  dimension "d365" = 2.5
  dimension "d366" = 4.5
  dimension "d367" = 5
  dimension "d368" = 5
  dimension "d369" = 5
  dimension "d370" = 5
  dimension "d371" = 5
  dimension "d372" = 5
  dimension "d373" = 5
  dimension "d374" = 5
  dimension "d375" = 5
  dimension "d376" = 5
  dimension "d377" = 5
  dimension "d378" = 5
  dimension "d379" = 5
  dimension "d380" = 5
  dimension "d381" = 5
  dimension "d382" = 5
  dimension "d383" = 5
  dimension "d384" = 5
  dimension "d385" = 5
  dimension "d386" = 5
  dimension "d387" = 5
  dimension "d388" = 5
  dimension "d389" = 5
  dimension "d390" = 2.5
  dimension "d391" = 4.5
  dimension "d392" = 2.5
  dimension "d393" = 4.5
  dimension "d394" = 2.5
  dimension "d395" = 4.5
  dimension "d396" = 0.15
  dimension "d397" = 18
  dimension "d398" = 0.15
  dimension "d399" = 2.5
  dimension "d400" = 4.5
  dimension "d401" = 0.15
  dimension "d402" = 0.15
  dimension "d403" = 2.5
  dimension "d404" = 4.5
  dimension "d405" = 2.5
  dimension "d406" = 4.5
  constraint coincident A0.centre A5.centre
  constraint horizontal L0
  constraint vertical L1
  constraint horizontal L2
  constraint vertical L3
  constraint horizontal L4
  constraint vertical L5
  constraint horizontal L6
  constraint vertical L7
  constraint horizontal L8
  constraint perpendicular L8 L9
  constraint parallel L8 L10
  constraint parallel L9 L11
  constraint horizontal L14
  constraint perpendicular L14 L15
  constraint parallel L14 L16
  constraint parallel L15 L17
  constraint concentric A0 A5
  constraint horizontal L24
  constraint perpendicular L24 L25
  constraint parallel L24 L26
  constraint parallel L25 L27
  constraint concentric A2 A10
  constraint concentric A2 A11
  constraint concentric A2 A12
  constraint horizontal L30
  constraint perpendicular L30 L31
  constraint parallel L30 L32
  constraint parallel L31 L33
  constraint coincident L34 P3
  constraint coincident L35 P3
  constraint concentric A1 A13
  constraint concentric A4 A14
  constraint concentric A3 A15
  constraint concentric A0 A16
  constraint concentric A17 A18
  constraint horizontal L40
  constraint perpendicular L40 L41
  constraint parallel L40 L42
  constraint parallel L41 L43
  constraint coincident L44 A0.centre
  constraint coincident L45 A0.centre
  constraint horizontal L46
  constraint vertical L47
  constraint horizontal L48
  constraint vertical L49
  constraint concentric A0 A20
  constraint concentric A15 A21
  constraint concentric A14 A22
  constraint concentric A1 A23
  constraint concentric A11 A24
  constraint horizontal L52
  constraint vertical L53
  constraint horizontal L54
  constraint vertical L55
  constraint horizontal L56
  constraint vertical L57
  constraint horizontal L58
  constraint vertical L59
  constraint horizontal L60
  constraint perpendicular L60 L61
  constraint parallel L60 L62
  constraint parallel L61 L63
  constraint horizontal L74
  constraint vertical L69
  constraint horizontal L68
  constraint vertical L71
  constraint horizontal L70
  constraint perpendicular L70 L73
  constraint parallel L70 L75
  constraint parallel L67 L73
  constraint horizontal L79
  constraint vertical L92
  constraint horizontal L85
  constraint vertical L83
  constraint horizontal L88
  constraint perpendicular L88 L90
  constraint parallel L81 L88
  constraint parallel L89 L90
  constraint horizontal L76
  constraint vertical L80
  constraint horizontal L91
  constraint vertical L87
  constraint horizontal L86
  constraint perpendicular L86 L94
  constraint parallel L84 L86
  constraint parallel L78 L94
  constraint horizontal L121
  constraint vertical L109
  constraint horizontal L126
  constraint vertical L110
  constraint horizontal L97
  constraint perpendicular L97 L103
  constraint parallel L97 L122
  constraint parallel L103 L105
  constraint horizontal L96
  constraint vertical L117
  constraint horizontal L115
  constraint vertical L129
  constraint horizontal L99
  constraint perpendicular L99 L130
  constraint parallel L98 L99
  constraint parallel L130 L132
  constraint horizontal L125
  constraint vertical L119
  constraint horizontal L111
  constraint vertical L112
  constraint horizontal L101
  constraint perpendicular L101 L127
  constraint parallel L101 L106
  constraint parallel L114 L127
  constraint horizontal L102
  constraint vertical L135
  constraint horizontal L134
  constraint vertical L131
  constraint horizontal L124
  constraint perpendicular L104 L124
  constraint parallel L118 L124
  constraint parallel L104 L128
  constraint horizontal L151
  constraint vertical L150
  constraint horizontal L206
  constraint vertical L157
  constraint horizontal L148
  constraint perpendicular L148 L202
  constraint parallel L148 L154
  constraint parallel L167 L202
  constraint horizontal L149
  constraint vertical L191
  constraint horizontal L153
  constraint vertical L158
  constraint horizontal L208
  constraint perpendicular L201 L208
  constraint parallel L192 L208
  constraint parallel L160 L201
  constraint horizontal L194
  constraint vertical L152
  constraint horizontal L207
  constraint vertical L177
  constraint horizontal L209
  constraint perpendicular L200 L209
  constraint parallel L209 L211
  constraint parallel L163 L200
  constraint horizontal L214
  constraint vertical L137
  constraint horizontal L155
  constraint vertical L162
  constraint horizontal L193
  constraint perpendicular L193 L199
  constraint parallel L193 L205
  constraint parallel L172 L199
  constraint horizontal L142
  constraint vertical L140
  constraint horizontal L185
  constraint vertical L159
  constraint horizontal L147
  constraint perpendicular L147 L198
  constraint parallel L147 L170
  constraint parallel L165 L198
  constraint horizontal L175
  constraint vertical L187
  constraint horizontal L141
  constraint vertical L166
  constraint horizontal L139
  constraint perpendicular L139 L196
  constraint parallel L139 L144
  constraint parallel L180 L196
  constraint horizontal L169
  constraint vertical L181
  constraint horizontal L145
  constraint vertical L178
  constraint horizontal L173
  constraint perpendicular L173 L195
  constraint parallel L173 L182
  constraint parallel L179 L195
  constraint horizontal L138
  constraint vertical L168
  constraint horizontal L176
  constraint vertical L164
  constraint horizontal L174
  constraint perpendicular L174 L197
  constraint parallel L174 L186
  constraint parallel L161 L197
  constraint horizontal L290
  constraint vertical L289
  constraint horizontal L278
  constraint vertical L239
  constraint horizontal L245
  constraint vertical L261
  constraint horizontal L297
  constraint vertical L272
  constraint horizontal L248
  constraint vertical L300
  constraint horizontal L264
  constraint vertical L238
  constraint horizontal L307
  constraint vertical L279
  constraint horizontal L244
  constraint vertical L243
  constraint horizontal L301
  constraint vertical L259
  constraint horizontal L286
  constraint vertical L270
  constraint horizontal L260
  constraint vertical L246
  constraint horizontal L288
  constraint vertical L235
  constraint horizontal L249
  constraint vertical L227
  constraint horizontal L247
  constraint vertical L236
  constraint horizontal L303
  constraint vertical L251
  constraint horizontal L295
  constraint vertical L242
  constraint horizontal L252
  constraint vertical L216
  constraint horizontal L271
  constraint vertical L268
  constraint horizontal L231
  constraint vertical L267
  constraint horizontal L314
  constraint vertical L275
  constraint horizontal L281
  constraint vertical L287
  constraint horizontal L313
  constraint vertical L273
  constraint horizontal L265
  constraint vertical L219
  constraint horizontal L220
  constraint vertical L266
  constraint horizontal L218
  constraint vertical L293
  constraint horizontal L222
  constraint vertical L237
  constraint horizontal L284
  constraint vertical L298
  constraint horizontal L228
  constraint vertical L240
  constraint horizontal L254
  constraint vertical L309
  constraint horizontal L292
  constraint vertical L234
  constraint horizontal L229
  constraint vertical L299
  constraint horizontal L223
  constraint vertical L241
  constraint vertical L316
  constraint concentric A25 A26
  constraint concentric A28 A29
  constraint vertical L318
  constraint parallel L36 L319
  constraint concentric A31 A33
  constraint concentric A37 A39
  constraint horizontal L364
  constraint horizontal L358
  constraint vertical L361
  constraint vertical L359
  constraint horizontal L369
  constraint horizontal L374
  constraint vertical L372
  constraint vertical L370
  constraint horizontal L381
  constraint vertical L384
  constraint vertical L382
  constraint horizontal L386
  constraint vertical L395
  constraint horizontal L392
  constraint vertical L394
  constraint horizontal L398
  constraint horizontal L409
  constraint horizontal L413
  constraint vertical L410
  constraint vertical L405
  constraint horizontal L422
  constraint vertical L424
  constraint horizontal L426
  constraint vertical L421
  constraint horizontal L433
  constraint vertical L435
  constraint vertical L434
  constraint horizontal L438
  constraint horizontal L446
  constraint horizontal L450
  constraint vertical L445
  constraint vertical L447
  constraint concentric A34 A36
  constraint concentric A43 A45
  constraint concentric A41 A42
  constraint vertical L453
  constraint horizontal L454
  constraint parallel L454 L497
  constraint parallel L454 L498
  constraint concentric A49 A50
  constraint concentric A55 A57
  constraint concentric A52 A54
  measures "d1" diameter of A0
  measures "d9" diameter of A1
  measures "d10" diameter of A2
  measures "d11" diameter of A3
  measures "d12" diameter of A4
  measures "d43" diameter of A6
  measures "d104" diameter of A10
  measures "d105" diameter of A11
  measures "d106" diameter of A12
  measures "d136" distance of L31.end L32.end
  measures "d137" distance of L30.end L31.end
  measures "d145" diameter of A13
  measures "d146" diameter of A14
  measures "d147" diameter of A15
  measures "d154" diameter of A16
  measures "d157" diameter of A17
  measures "d158" diameter of A18
  measures "d159" distance of L41.end L42.end
  measures "d160" distance of L40.end L41.end
  measures "d161" distance of L40.start L40.end
  measures "d162" distance of L40.start L48.end
  measures "d184" diameter of A21
  measures "d187" diameter of A22
  measures "d188" diameter of A23
  measures "d189" diameter of A24
  measures "d215" distance of L56.start L56.end
  measures "d216" distance of L56.start L58.end
  measures "d221" distance of L56.start L56.end
  measures "d222" distance of L56.start L58.end
  measures "d225" distance of L76.start L76.end
  measures "d226" distance of L76.start L83.start
  measures "d229" distance of L76.end L76.start
  measures "d230" distance of L76.start L83.start
  measures "d233" distance of L96.start L96.end
  measures "d234" distance of L96.start L110.start
  measures "d237" distance of L96.end L96.start
  measures "d238" distance of L96.start L110.start
  measures "d241" distance of L102.start L102.end
  measures "d242" distance of L102.start L111.end
  measures "d245" distance of L102.start L102.end
  measures "d246" distance of L102.start L111.end
  measures "d249" distance of L149.start L149.end
  measures "d250" distance of L149.start L153.end
  measures "d253" distance of L149.end L149.start
  measures "d254" distance of L149.start L153.end
  measures "d257" distance of L162.end L137.start
  measures "d258" distance of L162.end L155.end
  measures "d261" distance of L162.end L137.start
  measures "d262" distance of L162.end L155.end
  measures "d265" distance of L140.start L142.start
  measures "d266" distance of L141.end L142.start
  measures "d269" distance of L140.start L142.start
  measures "d270" distance of L141.end L142.start
  measures "d273" distance of L138.end L138.start
  measures "d274" distance of L138.start L145.end
  measures "d277" distance of L138.end L138.start
  measures "d278" distance of L145.end L138.start
  measures "d348" diameter of A26
  measures "d349" diameter of A25
  measures "d352" diameter of A28
  measures "d353" diameter of A29
  measures "d357" diameter of A31
  measures "d358" diameter of A33
  measures "d365" diameter of A39
  measures "d366" diameter of A37
  measures "d390" diameter of A34
  measures "d391" diameter of A36
  measures "d392" diameter of A45
  measures "d393" diameter of A43
  measures "d394" diameter of A41
  measures "d395" diameter of A42
  measures "d399" diameter of A50
  measures "d400" diameter of A49
  measures "d403" diameter of A55
  measures "d404" diameter of A57
  measures "d405" diameter of A52
  measures "d406" diameter of A54
sketch "Shell" plane through (0, 0, 0) normal (0, 1, 0) x (1, 0, 0)
  circle A0 centre (0, 0) radius 54.083269
  circle A1 centre (0, 0) radius 56.083269
  dimension "d29" = 2
  constraint coincident A0.centre A1.centre
extrude "Extrude6" add sketch "Shell" along normal blind 30 makes body 1
extrude "Extrude7" add sketch "Shell" along normal blind 2 contours A0 picked at (6.427646, -1.832679) bodies 1
extrude "Extrude8" add sketch "Blueprint" along normal blind 30 separate body contours L9 L10 L11 A5 picked at (-1.233383, 60.560963) makes body 2